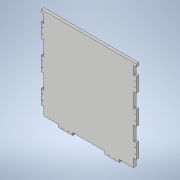
# Autodesk Inventor part: bottom-tool_part
Saved by Autodesk Inventor 2020 (Build 240168000, 168)
## iProperties
Created: 2019-12-17
Part Number: bottom-tool_part
Material: Generic
Document SubType Name: Modeling
Designer: fabfarm
Density: 1 g/cm^3
Appearance: Default
Author: fabfarm
Autodesk Inventor part; units mm, degrees
ref_plane "YZ Plane" through (0, 0, 0) normal (1, 0, 0) x (0, 1, 0)
ref_plane "XZ Plane" through (0, 0, 0) normal (0, 1, 0) x (-1, 0, 0)
ref_plane "XY Plane" through (0, 0, 0) normal (0, 0, 1) x (1, 0, 0)
sketch "Sketch1" plane through (0, 0, 0) normal (0, 0, 1) x (1, 0, 0)
  line L0 (330, -307.45) -> (-330, -307.45)
  line L1 (-330, -307.45) -> (-330, 307.45)
  line L2 (-330, 307.45) -> (330, 307.45)
  line L3 (330, 307.45) -> (330, -307.45)
  line L4 (330, -307.45) -> (-330, 307.45) construction
  line L5 (-330, -307.45) -> (330, 307.45) construction
  point P0 (0, 0)
  dimension "d0" = 614.9
  dimension "d1" = 660
  constraints: 12 end point, 2 midpoint, 2 parallel, 1 horizontal, 1 perpendicular
  measures "d0" distance of L2.end L0.start
  measures "d1" distance of L0.start L0.end
extrude "Extrusion1" add sketch "Sketch1" along normal blind 18.55
sketch "Sketch2" plane through (0, 0, 18.55) normal (0, 0, 1) x (1, 0, 0)
  line L0 (-330, 307.45) -> (-330, -307.45) construction
  line L1 (330, 307.45) -> (-330, 307.45) construction
  line L2 (-330, 307.45) -> (-311.45, 307.45)
  line L3 (-311.45, 307.45) -> (-311.45, 249.85)
  line L4 (-311.45, 249.85) -> (-330, 249.85)
  line L5 (-330, 249.85) -> (-330, 307.45)
  line L6 (-330, -307.45) -> (330, -307.45) projected
  line L7 (-330, -307.45) -> (-311.45, -307.45)
  line L8 (-311.45, -307.45) -> (-311.45, -249.85)
  line L9 (-311.45, -249.85) -> (-330, -249.85)
  line L10 (-330, -249.85) -> (-330, -307.45)
  line L11 (-330, -150.15) -> (-311.45, -150.15)
  line L12 (-311.45, -150.15) -> (-311.45, -49.95)
  line L13 (-311.45, -49.95) -> (-330, -49.95)
  line L14 (-330, -49.95) -> (-330, -150.15)
  line L15 (-330, 49.85) -> (-311.45, 49.85)
  line L16 (-311.45, 49.85) -> (-311.45, 150.05)
  line L17 (-311.45, 150.05) -> (-330, 150.05)
  line L18 (-330, 150.05) -> (-330, 49.85)
  point P0 (0, 0)
  dimension "d21" = 99.8
  dimension "d22" = 100.2
  dimension "d23" = 99.8
  dimension "d24" = 100.2
  dimension "d25" = 57.6
  dimension "d26" = 18.55
  dimension "d30" = 99.7
  constraints: 32 end point, 8 parallel, 5 point on line, 4 horizontal, 4 perpendicular, 3 collinear
  measures "d21" distance between parallel lines of L4 L17
  measures "d22" distance of L15.end L16.end
  measures "d23" distance between parallel lines of L13 L15
  measures "d24" distance of L11.end L12.end
  measures "d25" distance of L2.end L3.end
  measures "d26" distance of L0.end L7.end
  measures "d30" distance between parallel lines of L11 L9
extrude "Extrusion2" cut sketch "Sketch2" against normal blind 18.55
mirror "Mirror1" about plane through (0, 0, 0) normal (1, 0, 0) of "Extrusion2"
sketch "Esquisse5" plane through (0, 0, 18.55) normal (0, 0, 1) x (1, 0, 0)
  circle A0 centre (-312.5743, 250.9743) radius 1.59
  circle A1 centre (-312.5743, 148.9257) radius 1.59
  circle A2 centre (-312.5743, 50.9743) radius 1.59
  circle A3 centre (-312.5743, -51.0743) radius 1.59
  circle A4 centre (-312.5743, -149.0257) radius 1.59
  circle A5 centre (-312.5743, -250.9743) radius 1.59
  line L0 (311.45, 307.45) -> (-311.45, 307.45) projected
  line L1 (0, 307.45) -> (0, -307.45) construction
  line L2 (-311.45, -307.45) -> (311.45, -307.45) projected
  circle A6 centre (312.5743, 250.9743) radius 1.59
  circle A7 centre (312.5743, 148.9257) radius 1.59
  circle A8 centre (312.5743, 50.9743) radius 1.59
  circle A9 centre (312.5743, -51.0743) radius 1.59
  circle A10 centre (312.5743, -149.0257) radius 1.59
  circle A11 centre (312.5743, -250.9743) radius 1.59
  line L3 (-312.5743, 250.9743) -> (-311.45, 249.85) construction
  line L4 (-311.45, 249.85) -> (-330, 249.85) projected
  point P0 (0, 0)
  point P1 (-330, 49.85)
  point P2 (-330, -49.95)
  point P3 (-311.45, -249.85)
  point P4 (-311.45, -150.15)
  point P5 (-311.45, -49.95)
  point P6 (-311.45, 49.85)
  point P7 (-311.45, 150.05)
  dimension "d27" = 3.18
  dimension "d57" = 45
  constraints: 6 centre point, 6 symmetric about line, 5 vertical alignment, 4 end point, 2 midpoint, 24 other
  measures "d57" angle of L3 L4
extrude "Extrusion5" cut sketch "Esquisse5" against normal blind 18.55
sketch "Esquisse7" plane through (0, 0, 18.55) normal (0, 0, 1) x (1, 0, 0)
  line L0 (-311.45, -307.45) -> (311.45, -307.45) projected
  line L1 (-211.45, -307.45) -> (-111.55, -307.45)
  line L2 (-111.55, -307.45) -> (-111.55, -326)
  line L3 (-111.55, -326) -> (-211.45, -326)
  line L4 (-211.45, -326) -> (-211.45, -307.45)
  line L5 (111.55, -307.45) -> (211.45, -307.45)
  line L6 (211.45, -307.45) -> (211.45, -326)
  line L7 (211.45, -326) -> (111.55, -326)
  line L8 (111.55, -326) -> (111.55, -307.45)
  line L9 (-311.45, -252.0986) -> (-311.45, -307.45) projected
  line L10 (311.45, -307.45) -> (311.45, -252.0986) projected
  line L11 (-330, 49.85) -> (-330, -49.95) projected
  line L12 (-330, -0.05) -> (330, -0.05) construction
  line L13 (330, -49.95) -> (330, 49.85) projected
  circle A0 centre (-181.45, -316.725) radius 2.25
  circle A1 centre (-141.55, -316.725) radius 2.25
  circle A2 centre (141.55, -316.725) radius 2.25
  circle A3 centre (181.45, -316.725) radius 2.25
  line L14 (-211.45, -316.725) -> (-111.55, -316.725) construction
  line L15 (311.45, 307.45) -> (-311.45, 307.45) projected
  line L16 (-311.45, 307.45) -> (311.45, 307.45)
  line L17 (311.45, 307.45) -> (311.45, 326)
  line L18 (311.45, 326) -> (-311.45, 326)
  line L19 (-311.45, 326) -> (-311.45, 307.45)
  line L20 (311.45, 252.0986) -> (311.45, 307.45) projected
  point P0 (0, 0)
  dimension "d41" = 99.9
  dimension "d42" = 99.9
  dimension "d43" = 100
  dimension "d44" = 100
  dimension "d45" = 18.55
  dimension "d46" = 4.5
  dimension "d47" = 30
  dimension "d48" = 30
  dimension "d49" = 30
  dimension "d50" = 30
  dimension "d56" = 18.55
  constraints: 28 end point, 7 point on line, 6 parallel, 4 centre point, 4 midpoint, 3 equal radius, 3 horizontal, 3 perpendicular, 1 collinear
  measures "d41" distance of L2.end L3.end
  measures "d42" distance of L6.end L7.end
  measures "d43" distance between parallel lines of L9 L4
  measures "d44" distance between parallel lines of L6 L10
  measures "d45" distance of L1.end L2.end
  measures "d46" diameter of A0
  measures "d47" distance from line of L4 A0.centre
  measures "d48" distance from line of L2 A1.centre
  measures "d49" distance from line of L8 A2.centre
  measures "d50" distance from line of L6 A3.centre
  measures "d56" distance between parallel lines of L18 L15
extrude "Extrusion7" add sketch "Esquisse7" against normal blind 18.55
sketch "Esquisse6" plane through (0, 0, 18.55) normal (0, 0, 1) x (1, 0, 0)
  line L0 (-321.8493, -49.95) -> (-321.8493, 49.85) construction
  line L1 (-313.6986, 49.85) -> (-330, 49.85) construction
  line L2 (-313.6986, 150.05) -> (-330, 150.05) construction
  line L3 (-313.6986, 249.85) -> (-330, 249.85) construction
  circle A0 centre (-321.8493, 219.85) radius 2.25
  line L4 (-330, -49.95) -> (-313.6986, -49.95) projected
  line L5 (-0.1695, -446.756) -> (0, 307.45) construction
  line L6 (311.45, 307.45) -> (-311.45, 307.45) projected
  line L7 (-321.8493, 150.05) -> (-321.8493, 249.85) construction
  circle A1 centre (-321.8493, 180.05) radius 2.25
  circle A2 centre (-321.8493, 19.85) radius 2.25
  circle A3 centre (-321.8493, -19.95) radius 2.25
  line L8 (-313.6986, -150.15) -> (-330, -150.15) projected
  line L9 (-321.8493, -150.15) -> (-321.8493, -249.85) construction
  line L10 (-313.6986, -249.85) -> (-330, -249.85) projected
  circle A4 centre (-321.8493, -180.15) radius 2.25
  circle A5 centre (-321.8493, -219.85) radius 2.25
  line L11 (321.6886, -50.0947) -> (321.7334, 49.7053) construction
  line L12 (313.5827, 49.709) -> (329.8841, 49.7017) construction
  line L13 (313.6278, 149.909) -> (329.9292, 149.9016) construction
  line L14 (313.6727, 249.709) -> (329.9741, 249.7016) construction
  circle A6 centre (321.8099, 219.7053) radius 2.25
  line L15 (329.8393, -50.0983) -> (313.5379, -50.091)
  line L16 (321.7785, 149.9053) -> (321.8234, 249.7053) construction
  circle A7 centre (321.792, 179.9053) radius 2.25
  circle A8 centre (321.72, 19.7053) radius 2.25
  circle A9 centre (321.7021, -20.0947) radius 2.25
  line L17 (313.4928, -150.291) -> (329.7942, -150.2983)
  line L18 (321.6435, -150.2947) -> (321.5987, -249.9946) construction
  line L19 (313.448, -249.991) -> (329.7494, -249.9983)
  circle A10 centre (321.63, -180.2947) radius 2.25
  circle A11 centre (321.6122, -219.9947) radius 2.25
  point P0 (0, 0)
  dimension "d34" = 30
  dimension "d35" = 30
  dimension "d36" = 30
  dimension "d37" = 30
  dimension "d38" = 4.5
  dimension "d39" = 30
  dimension "d40" = 30
  constraints: 26 end point, 24 symmetric about line, 12 centre point, 12 point on line, 8 midpoint, 5 equal radius, 1 vertical, 6 other
  measures "d34" distance from line of L3 A0.centre
  measures "d35" distance from line of L2 A1.centre
  measures "d36" distance from line of L4 A3.centre
  measures "d37" distance from line of L1 A2.centre
  measures "d38" diameter of A0
  measures "d39" distance from line of L10 A5.centre
  measures "d40" distance from line of L8 A4.centre
extrude "Extrusion6" cut sketch "Esquisse6" against normal blind 20
sketch "Esquisse8" plane through (0, 0, 18.55) normal (0, 0, 1) x (1, 0, 0)
  circle A0 centre (-212.5814, -308.5814) radius 1.6
  circle A1 centre (-110.4186, -308.5814) radius 1.6
  circle A2 centre (110.4186, -308.5814) radius 1.6
  circle A3 centre (212.5814, -308.5814) radius 1.6
  line L0 (211.45, -307.45) -> (212.5814, -308.5814) construction
  line L1 (211.45, -307.45) -> (311.45, -307.45) projected
  point P0 (0, 0)
  point P1 (-111.55, -307.45)
  point P2 (-211.45, -307.45)
  point P3 (111.55, -307.45)
  dimension "d53" = 3.2
  dimension "d58" = 45
  constraints: 3 horizontal alignment, 2 end point, 12 other
  measures "d58" angle of L1 L0
extrude "Extrusion8" cut sketch "Esquisse8" against normal blind 18.55
sketch "Esquisse10" plane through (0, 0, 18.55) normal (0, 0, 1) x (1, 0, 0)
  line L0 (-311.45, 326) -> (-311.45, 252.0986) projected
  line L1 (-311.45, 326) -> (-330, 326)
  line L2 (-330, 326) -> (-330, 307.55)
  line L3 (-330, 307.55) -> (-311.45, 307.55)
  line L4 (-311.45, 307.55) -> (-311.45, 326)
  line L5 (311.45, 326) -> (-311.45, 326) projected
  line L6 (311.45, 326) -> (330, 326)
  line L7 (330, 326) -> (330, 307.55)
  line L8 (330, 307.55) -> (311.45, 307.55)
  line L9 (311.45, 307.55) -> (311.45, 326)
  line L10 (330, 150.05) -> (330, 249.85) projected
  line L11 (-330, 249.85) -> (-330, 150.05) projected
  point P0 (0, 0)
  dimension "d59" = 18.45
  constraints: 16 end point, 4 parallel, 2 collinear, 2 horizontal, 2 perpendicular, 1 point on line
  measures "d59" distance of L6.end L7.end
extrude "Extrusion9" add sketch "Esquisse10" against normal blind 18.55
sketch "Esquisse11" plane through (0, 0, 18.55) normal (0, 0, 1) x (1, 0, 0)
  line L0 (-311.45, 307.55) -> (-311.45, 252.0986) projected
  circle A0 centre (-312.5814, 306.4186) radius 1.6
  line L1 (311.45, 252.0986) -> (311.45, 307.55) projected
  circle A1 centre (312.5814, 306.4186) radius 1.6
  line L2 (311.45, 307.55) -> (312.5814, 306.4186) construction
  point P0 (0, 0)
  dimension "d63" = 3.2
  dimension "d62" = 45
  constraints: 2 end point, 1 horizontal alignment, 6 other
  measures "d62" angle of L1 L2
extrude "Extrusion10" cut sketch "Esquisse11" against normal blind 20
body "Solid1"
